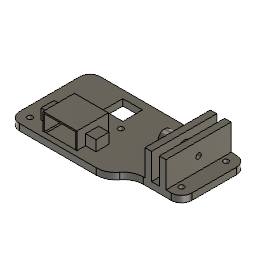
payload drop mechanism (Autodesk Fusion 360 design; units mm, degrees)
part number: 2026-04-05-16-47-29-307
Autodesk Fusion 360 part; units mm, degrees
sketch "Sketch1" plane through (0, 0, 0) normal (0, 0, 1) x (1, 0, 0)
  line L0 (0, 0) -> (120, 0)
  line L1 (120, 0) -> (120, 50)
  line L2 (120, 50) -> (0, 50)
  line L3 (0, 50) -> (0, 0)
  dimension "d1" = 120
  dimension "d2" = 50
  constraint horizontal L0
  constraint vertical L1
  constraint horizontal L2
  constraint vertical L3
  constraint coincident L0.start L3.end
  measures "d1" distance of L0.start L0.end
  measures "d2" distance of L0.start L2.end
extrude "Extrude1" add sketch "Sketch1" along normal blind 5 makes body 1
sketch "Sketch2" plane through (0, 0, 0) normal (0, 0, 1) x (1, 0, 0)
  line L0 (0, 0) -> (76, 0)
  line L1 (76, 0) -> (76, -12)
  line L2 (76, -12) -> (0, -12)
  line L3 (0, -12) -> (0, 0)
  dimension "d5" = 76
  dimension "d6" = 12
  constraint horizontal L0
  constraint vertical L1
  constraint horizontal L2
  constraint vertical L3
  constraint coincident L0.start L3.end
  measures "d5" distance of L0.start L0.end
  measures "d6" distance of L0.start L2.end
extrude "Extrude2" add sketch "Sketch2" along normal blind 5 bodies 1
fillet "Fillet1" radius 15 1 edges at (76, 0, 2.5) on bodies 1
fillet "Fillet2" radius 15 1 edges at (76, -12, 2.5) on bodies 1
fillet "Fillet3" radius 8 2 edges at (0, -12, 2.5) (0, 50, 2.5) on bodies 1
sketch "Sketch3" plane through (0, 0, 0) normal (0, 0, 1) x (1, 0, 0)
  line L0 (0, -12) -> (8, -12) construction
  line L1 (8, -12) -> (8, -4) construction
  line L2 (8, -4) -> (0, -4) construction
  line L3 (0, -4) -> (0, -12) construction
  circle A0 centre (8, -4) radius 2
  circle A1 centre (8, 42) radius 2
  circle A2 centre (112, 42) radius 2
  line L4 (120, 50) -> (120, 0)
  line L5 (120, 25) -> (108.8179, 25)
  circle A3 centre (112, 8) radius 2
  point P0 (9, -12)
  point P1 (0, -12)
  dimension "d15" = 8
  dimension "d16" = 8
  dimension "d17" = 4
  constraint horizontal L0
  constraint vertical L1
  constraint horizontal L2
  constraint vertical L3
  constraint coincident P1 L0.start
  constraint coincident L1.end L2.start
  constraint vertical L4
  constraint midpoint L4 L5.start
  constraint perpendicular L4 L5
  constraint symmetric A2 L5 A3
  measures "d15" distance of P1 L0.end
  measures "d16" distance of P1 L2.end
  measures "d17" diameter of A0
fillet "Fillet4" radius 8 2 edges at (120, 0, 2.5) (120, 50, 2.5) on bodies 1
extrude "Extrude3" cut sketch "Sketch3" along normal blind 20 bodies 1
sketch "Sketch4" plane through (0, 0, 5) normal (0, 0, 1) x (-1, 0, 0)
  circle A0 centre (-8, 4) radius 2
  circle A1 centre (-112, -42) radius 2
  circle A2 centre (-8, -42) radius 2
  circle A3 centre (-112, -8) radius 2
  arc A4 (-120, -42) -> (-112, -50) centre (-112, -42) ccw
  line L0 (-112, -50) -> (-8, -50)
  arc A5 (-8, -50) -> (0, -42) centre (-8, -42) ccw
  line L1 (0, -42) -> (0, 4)
  arc A6 (0, 4) -> (-8, 12) centre (-8, 4) ccw
  line L2 (-8, 12) -> (-66.6969, 12)
  arc A7 (-66.6969, 12) -> (-78.6969, 6) centre (-66.6969, -3) ccw
  arc A8 (-90.6969, 0) -> (-78.6969, 6) centre (-90.6969, 15) ccw
  line L3 (-90.6969, 0) -> (-112, 0)
  arc A9 (-112, 0) -> (-120, -8) centre (-112, -8) ccw
  line L4 (-120, -8) -> (-120, -42)
  line L5 (-31.0589, -44) -> (-46.0589, -44)
  line L6 (-46.0589, -44) -> (-46.0589, -29)
  line L7 (-46.0589, -29) -> (-31.0589, -29)
  line L8 (-31.0589, -29) -> (-31.0589, -44)
  line L9 (-38.5589, -44) -> (-38.5589, -29) construction
  circle A10 centre (-26.8349, -23.3563) radius 2
  circle A11 centre (-50.2829, -23.3563) radius 2
  point P0 (-8, -44)
  dimension "d22" = 15
  dimension "d23" = 15
  dimension "d24" = 4
  constraint coincident A2 P0
  constraint horizontal L5
  constraint vertical L6
  constraint horizontal L7
  constraint vertical L8
  constraint midpoint L5 L9.start
  constraint midpoint L7 L9.end
  constraint symmetric L9 A10 A11
  measures "d22" distance of L5.start L5.end
  measures "d23" distance of L5.start L7.end
  measures "d24" diameter of A10
extrude "Extrude4" cut sketch "Sketch4" against normal blind 140 contours L5 L6 L7 L8 | A10 | A11 bodies 1
sketch "Sketch5" plane through (0, 0, 5) normal (0, 0, 1) x (-1, 0, 0)
  line L0 (-46.0589, -44) -> (-46.0589, -29)
  line L1 (-46.0589, -29) -> (-31.0589, -29)
  line L2 (-31.0589, -29) -> (-31.0589, -44)
  line L3 (-31.0589, -44) -> (-46.0589, -44)
  circle A0 centre (-26.8349, -23.3563) radius 2
  circle A1 centre (-50.2829, -23.3563) radius 2
  circle A2 centre (-8, 4) radius 2
  circle A3 centre (-112, -42) radius 2
  circle A4 centre (-8, -42) radius 2
  circle A5 centre (-112, -8) radius 2
  arc A6 (-120, -42) -> (-112, -50) centre (-112, -42) ccw
  line L4 (-112, -50) -> (-8, -50)
  arc A7 (-8, -50) -> (0, -42) centre (-8, -42) ccw
  line L5 (0, -42) -> (0, 4)
  arc A8 (0, 4) -> (-8, 12) centre (-8, 4) ccw
  line L6 (-8, 12) -> (-66.6969, 12)
  arc A9 (-66.6969, 12) -> (-78.6969, 6) centre (-66.6969, -3) ccw
  arc A10 (-90.6969, 0) -> (-78.6969, 6) centre (-90.6969, 15) ccw
  line L7 (-90.6969, 0) -> (-112, 0)
  arc A11 (-112, 0) -> (-120, -8) centre (-112, -8) ccw
  line L8 (-120, -8) -> (-120, -42)
  line L9 (0, -20) -> (-8, -20)
  line L10 (-8, -20) -> (-8, -28)
  line L11 (-6, -30) -> (0, -30)
  line L12 (0, -30) -> (0, -20)
  line L13 (-8, -28) -> (-6, -30)
  line L14 (-7, -36) -> (3, -36) construction
  line L15 (-7, -36) -> (-8.7678, -37.7678)
  line L16 (-15.8388, -30.6967) -> (-14.0711, -28.9289)
  line L17 (-14.0711, -28.9289) -> (-13.0104, -29.9896)
  line L18 (-13.0104, -29.9896) -> (-14.7782, -31.7574)
  line L19 (-7, -36) -> (-8.0607, -34.9393)
  line L20 (-8.0607, -34.9393) -> (-9.8284, -36.7071)
  line L21 (-7, -36) -> (-8.0607, -34.9393)
  line L22 (-13.0104, -29.9896) -> (-14.0711, -28.9289)
  line L23 (-8.7678, -37.7678) -> (-9.8284, -36.7071)
  line L24 (-14.7782, -31.7574) -> (-15.8388, -30.6967)
  point P0 (-8, -30)
  dimension "d27" = 8
  dimension "d28" = 10
  dimension "d29" = 2
  dimension "d30" = 2
  dimension "d31" = 135
  dimension "d32" = 10
  dimension "d33" = 2.5
  dimension "d34" = 10
  dimension "d35" = 1.5
  dimension "d36" = 1.5
  constraint horizontal L9
  constraint vertical L10
  constraint horizontal L11
  constraint vertical L12
  constraint coincident L5 L9.start
  constraint coincident P0 L10
  constraint coincident P0 L11
  constraint horizontal L14
  constraint perpendicular L15 L21
  constraint perpendicular L15 L23
  constraint perpendicular L16 L17
  constraint perpendicular L18 L24
  constraint perpendicular L15 L19
  constraint perpendicular L20 L23
  constraint collinear L21 L22
  constraint collinear L23 L24
  measures "d27" distance of L9.start L9.end
  measures "d28" distance of L9.start L11.end
  measures "d29" distance of P0 L10.end
  measures "d30" distance of P0 L11.start
  measures "d31" angle of L14 L21
  measures "d32" distance of L14.start L16.end
  measures "d33" distance of L14.start L15.end
  measures "d34" distance of L15.end L16.start
  measures "d35" distance of L16.end L17.end
  measures "d36" distance of L14.start L19.end
extrude "Extrude5" add sketch "Sketch5" against normal blind 5 contours A4 bodies 1
extrude "Extrude6" add sketch "Sketch5" along normal blind 10 contours L5 L9 L10 L11 L12 L13 | L15 L19 L20 L21 L23 | L16 L17 L18 L22 L24 bodies 1
sketch "Sketch6" plane through (0, 0, 15) normal (0, 0, 1) x (-1, 0, 0)
  line L0 (-7, -36) -> (-8.0607, -34.9393)
  line L1 (-8.0607, -34.9393) -> (-9.8284, -36.7071)
  line L2 (-9.8284, -36.7071) -> (-8.7678, -37.7678)
  line L3 (-8.7678, -37.7678) -> (-7, -36)
  line L4 (-7, -36) -> (-14.0711, -28.9289)
  line L5 (-7, -36) -> (-8.7678, -37.7678)
  line L6 (-8.7678, -37.7678) -> (-15.8388, -30.6967)
  line L7 (-15.8388, -30.6967) -> (-14.0711, -28.9289)
  dimension "d41" = 10
  dimension "d42" = 10
  constraint coincident L0.start L3.end
  constraint perpendicular L3 L4
  constraint coincident L2.end L3.start
  constraint perpendicular L1 L6
  measures "d41" distance of L0.start L4.end
  measures "d42" distance of L2.end L6.end
delete_face "DeleteFace1" 1 faces at (13.7175, 29.2825, 8.3333) on bodies 1
delete_face "DeleteFace2" 1 faces at (7.3536, 35.6464, 8.3333) on bodies 1
extrude "Extrude7" add sketch "Sketch5" along normal blind 7 contours L15 L19 L20 L21 L23 | L16 L17 L18 L22 L24 bodies 1
extrude "Extrude8" add sketch "Sketch6" against normal blind 3 bodies 1
sketch "Sketch7" plane through (0, 0, 5) normal (0, 0, 1) x (-1, 0, 0)
  line L0 (-22, -15) -> (-48, -15) construction
  line L1 (-48, -15) -> (-48, 8) construction
  line L2 (-48, 8) -> (-22, 8) construction
  line L3 (-22, 8) -> (-22, -15) construction
  line L4 (-35, -15) -> (-35, 8) construction
  line L5 (-22, -3.5) -> (-48, -3.5) construction
  line L6 (-22, -8.5) -> (-14, -8.5)
  line L7 (-14, -8.5) -> (-14, 1.5)
  line L8 (-14, 1.5) -> (-22, 1.5)
  line L9 (-30, -8.5) -> (-14, 1.5) construction
  line L10 (-14, -8.5) -> (-30, 1.5) construction
  line L11 (-22, -8.5) -> (-22, 1.5)
  line L12 (-48, -8.5) -> (-56, -8.5)
  line L13 (-56, -8.5) -> (-56, 1.5)
  line L14 (-56, 1.5) -> (-48, 1.5)
  line L15 (-48, -8.5) -> (-48, 1.5)
  line L16 (-22, -15) -> (-48, -15)
  line L17 (-48, -15) -> (-48, 8)
  line L18 (-48, 8) -> (-22, 8)
  line L19 (-22, 8) -> (-22, -15)
  point P0 (-22, -3.5)
  dimension "d47" = 26
  dimension "d48" = 23
  dimension "d49" = 16
  dimension "d50" = 10
  constraint horizontal L0
  constraint vertical L1
  constraint horizontal L2
  constraint vertical L3
  constraint midpoint L0 L4.start
  constraint midpoint L2 L4.end
  constraint midpoint L3 P0
  constraint midpoint L1 L5.end
  constraint horizontal L6
  constraint perpendicular L6 L7
  constraint parallel L6 L8
  constraint coincident L9 P0
  constraint coincident L10 P0
  constraint coincident P0 L5.start
  constraint symmetric L4 L6.end L12.end
  constraint symmetric L4 L7.end L13.end
  constraint symmetric L4 L6.start L12.start
  constraint symmetric L4 L8.end L14.end
  constraint horizontal L16
  constraint vertical L17
  constraint horizontal L18
  constraint vertical L19
  measures "d47" distance of L0.start L0.end
  measures "d48" distance of L0.start L2.end
  measures "d49" distance of L7.end L10.end
  measures "d50" distance of L6.end L7.end
extrude "Extrude9" add sketch "Sketch7" along normal blind 8 contours L6 L7 L8 L11 L19 | L12 L13 L14 L15 L17 bodies 1
sketch "Sketch8" plane through (0, 0, 5) normal (0, 0, 1) x (-1, 0, 0)
  line L0 (-90.6969, 0) -> (-112, 0)
  line L1 (-108, -50) -> (-103, -50)
  line L2 (-103, -50) -> (-103, 0)
  line L3 (-103, 0) -> (-108, 0)
  line L4 (-108, 0) -> (-108, -50)
  line L5 (-97, -50) -> (-92, -50)
  line L6 (-92, -50) -> (-92, 0)
  line L7 (-92, 0) -> (-97, 0)
  line L8 (-97, 0) -> (-97, -50)
  dimension "d53" = 5
  dimension "d54" = 5
  dimension "d55" = 6
  constraint horizontal L1
  constraint vertical L2
  constraint horizontal L3
  constraint vertical L4
  constraint coincident L0 L2.end
  constraint horizontal L5
  constraint vertical L6
  constraint horizontal L7
  constraint vertical L8
  constraint coincident L0 L6.end
  measures "d53" distance of L1.start L1.end
  measures "d54" distance of L5.start L5.end
  measures "d55" distance of L2 L8
extrude "Extrude10" add sketch "Sketch8" along normal blind 20 bodies 1
sketch "Sketch9" plane through (97, 0, 0) normal (1, 0, 0) x (0, 1, 0)
  line L0 (0, 5) -> (50, 5)
  line L1 (50, 5) -> (50, 25)
  line L2 (50, 25) -> (0, 25)
  line L3 (0, 25) -> (0, 5)
  line L4 (0, 5) -> (50, 25) construction
  circle A0 centre (25, 15) radius 5
  dimension "d58" = 10
  constraint coincident L0.start L3.end
  constraint coincident L1.end L2.start
  constraint midpoint L4 A0.centre
  measures "d58" diameter of A0
extrude "Extrude11" add sketch "Sketch9" along normal blind 6 separate body contours A0 makes body 2
sketch "Sketch10" plane through (103, 0, 0) normal (1, 0, 0) x (0, 1, 0)
  circle A0 centre (25, 15) radius 5
  circle A1 centre (25, 15) radius 2
  dimension "d61" = 4
  constraint concentric A0 A1
  measures "d61" diameter of A1
extrude "Extrude12" cut sketch "Sketch10" along normal blind 13 and the other way blind 34 contours A1 bodies 1 2
extrude "Extrude13" add sketch "Sketch9" against normal blind 15 contours A0 bodies 1 2
sketch "Sketch11" plane through (0, 0, 5) normal (0, 0, 1) x (-1, 0, 0)
  line L0 (-75, -50) -> (-83, -50)
  line L1 (-83, -50) -> (-83, -42)
  line L2 (-83, -42) -> (-75, -42)
  line L3 (-75, -42) -> (-75, -50)
  line L4 (-92, -1) -> (-84, -1)
  line L5 (-84, -1) -> (-84, -9)
  line L6 (-84, -9) -> (-92, -9)
  line L7 (-92, -9) -> (-92, -1)
  dimension "d68" = 8
  dimension "d69" = 8
  dimension "d70" = 8
  dimension "d71" = 8
  constraint horizontal L0
  constraint vertical L1
  constraint horizontal L2
  constraint vertical L3
  constraint horizontal L4
  constraint vertical L5
  constraint horizontal L6
  constraint vertical L7
  measures "d68" distance of L0.start L0.end
  measures "d69" distance of L0.start L2.end
  measures "d70" distance of L4.start L4.end
  measures "d71" distance of L4.start L6.end
extrude "Extrude14" add sketch "Sketch11" along normal blind 4 bodies 1
extrude "Extrude15" cut sketch "Sketch7" against normal blind 2.5 contours L11 L15 L16 L17 L18 L19 bodies 1
sketch "Sketch12" plane through (0, 0, 5) normal (0, 0, 1) x (-1, 0, 0)
  line L0 (-48, -15) -> (-48, -8.5)
  line L1 (-48, -8.5) -> (-56, -8.5)
  line L2 (-56, -8.5) -> (-56, 1.5)
  line L3 (-56, 1.5) -> (-48, 1.5)
  line L4 (-48, 1.5) -> (-48, 8)
  line L5 (-48, 8) -> (-22, 8)
  line L6 (-22, 8) -> (-22, 1.5)
  line L7 (-22, 1.5) -> (-14, 1.5)
  line L8 (-14, 1.5) -> (-14, -8.5)
  line L9 (-14, -8.5) -> (-22, -8.5)
  line L10 (-22, -8.5) -> (-22, -15)
  line L11 (-22, -15) -> (-48, -15)
  line L12 (-92, -1) -> (-84, -1)
  line L13 (-84, -1) -> (-84, -9)
  line L14 (-84, -9) -> (-92, -9)
  line L15 (-92, -9) -> (-92, -50)
  line L16 (-92, -50) -> (-83, -50)
  line L17 (-83, -50) -> (-83, -42)
  line L18 (-83, -42) -> (-75, -42)
  line L19 (-75, -42) -> (-75, -50)
  line L20 (-75, -50) -> (-8, -50)
  arc A0 (-8, -50) -> (0, -42) centre (-8, -42) ccw
  line L21 (0, -42) -> (0, -30)
  line L22 (0, -30) -> (-6, -30)
  line L23 (-6, -30) -> (-8, -28)
  line L24 (-8, -28) -> (-8, -20)
  line L25 (-8, -20) -> (0, -20)
  line L26 (0, -20) -> (0, 4)
  arc A1 (0, 4) -> (-8, 12) centre (-8, 4) ccw
  line L27 (-8, 12) -> (-66.6969, 12)
  arc A2 (-66.6969, 12) -> (-78.6969, 6) centre (-66.6969, -3) ccw
  arc A3 (-90.6969, 0) -> (-78.6969, 6) centre (-90.6969, 15) ccw
  line L28 (-90.6969, 0) -> (-92, 0)
  line L29 (-92, 0) -> (-92, -1)
  line L30 (-7, -36) -> (-8.7678, -37.7678)
  line L31 (-8.7678, -37.7678) -> (-9.8284, -36.7071)
  line L32 (-9.8284, -36.7071) -> (-8.0607, -34.9393)
  line L33 (-8.0607, -34.9393) -> (-7, -36)
  line L34 (-13.0104, -29.9896) -> (-14.7782, -31.7574)
  line L35 (-14.7782, -31.7574) -> (-15.8388, -30.6967)
  line L36 (-15.8388, -30.6967) -> (-14.0711, -28.9289)
  line L37 (-14.0711, -28.9289) -> (-13.0104, -29.9896)
  circle A4 centre (-8, 4) radius 2
  circle A5 centre (-50.2829, -23.3563) radius 2
  circle A6 centre (-26.8349, -23.3563) radius 2
  line L38 (-46.0589, -44) -> (-46.0589, -29)
  line L39 (-46.0589, -29) -> (-31.0589, -29)
  line L40 (-31.0589, -29) -> (-31.0589, -44)
  line L41 (-31.0589, -44) -> (-46.0589, -44)
  line L42 (-22, -15) -> (-22, -16)
  line L43 (-22, -16) -> (-24, -16)
  line L44 (-24, -16) -> (-24, -15)
  line L45 (-24, -16) -> (-32, -16) construction
  line L46 (-32, -16) -> (-32, -15)
  line L47 (-32, -15) -> (-47, -15)
  line L48 (-48, -15) -> (-48, -16)
  line L49 (-48, -16) -> (-32, -16)
  line L50 (-22, -16) -> (-22, 8)
  line L51 (-23, 8) -> (-23, -15)
  line L52 (-22, 8) -> (-22, 9) construction
  line L53 (-48, 9) -> (-48, 8)
  line L54 (-22, 8) -> (-22, 9)
  line L55 (-47, 8) -> (-47, -15)
  line L56 (-47, -16) -> (-48, -16)
  line L57 (-48, -16) -> (-48, 8)
  line L58 (-22, -15) -> (-24, -15)
  line L59 (-22, 8) -> (-23, 8)
  line L60 (-47, 8) -> (-48, 8)
  dimension "d76" = 1
  dimension "d77" = 2
  dimension "d78" = 8
  dimension "d79" = 1
  dimension "d80" = 1
  dimension "d81" = 1
  constraint coincident L10.end L11.start
  constraint perpendicular L11 L42
  constraint perpendicular L42 L43
  constraint coincident L11 L44.end
  constraint perpendicular L11 L44
  constraint perpendicular L44 L45
  constraint coincident L11 L46.end
  constraint perpendicular L11 L46
  constraint coincident L0.start L11.end
  constraint perpendicular L11 L48
  constraint perpendicular L46 L49
  constraint coincident L5.end L6.start
  constraint perpendicular L5 L52
  constraint vertical L53
  constraint vertical L54
  constraint coincident L4.end L5.start
  constraint vertical L55
  constraint horizontal L56
  constraint vertical L57
  constraint coincident L11 L51.end
  constraint coincident L11 L47.end
  constraint perpendicular L51 L59
  constraint perpendicular L53 L60
  measures "d76" distance of L10.end L42.end
  measures "d77" distance of L42.end L43.end
  measures "d78" distance of L43.end L45.end
  measures "d79" distance of L5.end L51.start
  measures "d80" distance of L5.end L52.end
  measures "d81" distance of L4.end L55.start
sketch "Sketch13" plane through (82, 0, 0) normal (-1, 0, 0) x (0, -1, 0)
  circle A0 centre (-25, 15) radius 5
  circle A1 centre (-25, 15) radius 2
  dimension "d84" = 4
  constraint concentric A0 A1
  measures "d84" diameter of A1
extrude "Extrude17" cut sketch "Sketch13" against normal blind 32 contours A1 bodies 1
extrude "Extrude18" add sketch "Sketch12" along normal blind 13 separate body contours L0 L4 L5 L11 L55 L57 L60 | L11 L46 L47 L48 L49 L56 L57 | L11 L42 L43 L44 L50 L58 | L5 L6 L10 L11 L50 L51 L58 L59 makes body 3 at (22, 0, 9.3333) makes body 4 at (48, 8, 13.6667)
sketch "Sketch14" plane through (0, 0, 18) normal (0, 0, 1) x (-1, 0, 0)
  line L0 (-22, -16) -> (-22, 8)
  line L1 (-22, 8) -> (-23, 8)
  line L2 (-23, 8) -> (-23, -15)
  line L3 (-23, -15) -> (-24, -15)
  line L4 (-24, -15) -> (-24, -16)
  line L5 (-24, -16) -> (-22, -16)
  line L6 (-22, -16) -> (-48, -16)
  line L7 (-48, -16) -> (-48, 8)
  line L8 (-48, 8) -> (-22, 8)
  line L9 (-22, 8) -> (-22, -16)
  constraint horizontal L6
  constraint vertical L7
  constraint horizontal L8
  constraint vertical L9
  constraint coincident L0.start L5.end
extrude "Extrude19" add sketch "Sketch14" against normal blind 1 contours L2 L3 L4 L6 L7 L8 bodies 3 4
sketch "Sketch15" plane through (0, 0, 18) normal (0, 0, 1) x (-1, 0, 0)
  line L0 (-22, -16) -> (-22, 8)
  line L1 (-22, 8) -> (-48, 8)
  line L2 (-48, 8) -> (-48, -16)
  line L3 (-48, -16) -> (-22, -16)
  line L4 (-22, -16) -> (-35, -16)
  line L5 (-35, -16) -> (-35, -15)
  line L6 (-35, -15) -> (-22, -15)
  line L7 (-22, -15) -> (-22, -16)
  dimension "d91" = 1
  constraint horizontal L4
  constraint vertical L5
  constraint horizontal L6
  constraint vertical L7
  constraint coincident L0.start L3.end
  measures "d91" distance of L0.start L6.end
extrude "Extrude20" add sketch "Sketch15" against normal blind 5 contours L0 L3 L4 L5 L6 L7 bodies 3
sketch "Sketch16" plane through (0, 0, 15) normal (0, 0, 1) x (-1, 0, 0)
  line L0 (-8, -28) -> (-6, -30)
  line L1 (-6, -30) -> (0, -30)
  line L2 (0, -30) -> (0, -20)
  line L3 (0, -20) -> (-8, -20)
  line L4 (-8, -20) -> (-8, -28)
extrude "Extrude21" cut sketch "Sketch16" against normal blind 10 bodies 1
sketch "Sketch17" plane through (0, 0, 9) normal (0, 0, 1) x (-1, 0, 0)
  line L0 (-75, -42) -> (-83, -42)
  line L1 (-83, -42) -> (-83, -50)
  line L2 (-83, -50) -> (-75, -50)
  line L3 (-75, -50) -> (-75, -42)
  line L4 (-92, -9) -> (-84, -9)
  line L5 (-84, -9) -> (-84, -1)
  line L6 (-84, -1) -> (-92, -1)
  line L7 (-92, -1) -> (-92, -9)
extrude "Extrude22" cut sketch "Sketch17" against normal blind 4 bodies 1
sketch "Sketch18" plane through (0, 0, 15) normal (0, 0, 1) x (-1, 0, 0)
  line L0 (-7, -36) -> (-14.0711, -28.9289)
  line L1 (-14.0711, -28.9289) -> (-15.8388, -30.6967)
  line L2 (-15.8388, -30.6967) -> (-8.7678, -37.7678)
  line L3 (-8.7678, -37.7678) -> (-7, -36)
extrude "Extrude23" cut sketch "Sketch18" against normal blind 10 bodies 1
equation "d30 = d29"
